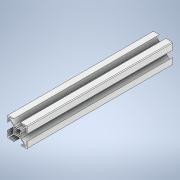
# Autodesk Inventor part: PerfilBaseJohan
Saved by Autodesk Inventor 2022.6 (Build 266554000, 554)
## iProperties
Created: 2025-01-14
Part Number: PerfilBaseJohan
Material: Genérico
Document SubType Name: Modeling
Designer: johan
Density: 1 g/cm^3
Appearance: Valor por defecto
Author: johan
Autodesk Inventor part; units mm, degrees
ref_plane "YZ Plane" through (0, 0, 0) normal (1, 0, 0) x (0, 1, 0)
ref_plane "XZ Plane" through (0, 0, 0) normal (0, 1, 0) x (-1, 0, 0)
ref_plane "XY Plane" through (0, 0, 0) normal (0, 0, 1) x (1, 0, 0)
sketch "Boceto1" plane through (0, 0, 0) normal (0, 0, 1) x (1, 0, 0)
  line L0 (0, 20) -> (7, 20)
  line L1 (7, 20) -> (7, 21)
  line L2 (0, 20) -> (1, 20)
  line L3 (1, 17.6407) -> (1, 15)
  line L4 (-1, 13) -> (0, 13)
  line L5 (5, 19) -> (2.3598, 19)
  arc A0 (5, 19) -> (6.7321, 20) centre (5, 21) ccw
  arc A1 (0, 13.2679) -> (1, 15) centre (-1, 15) ccw
  line L6 (20, 20) -> (13, 20)
  line L7 (19.3, 20) -> (19, 20)
  line L8 (19, 17.6402) -> (19, 15)
  line L9 (21, 13) -> (20, 13)
  line L10 (13, 20) -> (13, 21)
  line L11 (15, 19) -> (18.365, 19)
  arc A2 (13.2679, 20) -> (15, 19) centre (15, 21) ccw
  arc A3 (19, 15) -> (20, 13.2679) centre (21, 15) ccw
  line L12 (0.7, 0) -> (7, 0)
  line L13 (-1, 8.6378) -> (0, 8.6378)
  line L14 (7, 0) -> (7, -1)
  line L15 (5, 1) -> (2.3593, 1)
  line L16 (19.3, 0) -> (13, 0)
  line L17 (13, 0) -> (13, -1)
  line L18 (15, 1) -> (17.6402, 1)
  line L19 (19, 5) -> (19, 2.3593)
  arc A4 (20, 6.7321) -> (19, 5) centre (21, 5) ccw
  arc A5 (15, 1) -> (13.2679, 0) centre (15, -1) ccw
  arc A6 (6.7321, 0) -> (5, 1) centre (5, -1) ccw
  line L20 (20, 20) -> (13, 20)
  line L21 (7, 20) -> (0.7, 20)
  line L22 (0, 19.3) -> (0, 13)
  line L23 (0, 6.4641) -> (0, 0.7)
  line L24 (20, 0.7) -> (20, 6.7321)
  line L25 (20, 13) -> (20, 19.3)
  line L26 (0, 0) -> (7, 0)
  line L27 (13, 0) -> (20, 0)
  line L28 (17.6407, 19) -> (17.365, 19)
  line L29 (17.8529, 18.4879) -> (13.565, 14.2)
  line L30 (18.4883, 17.8528) -> (14.2, 13.5832)
  line L31 (1.5121, 17.8529) -> (5.8, 13.565)
  line L32 (2.1472, 18.4883) -> (6.4168, 14.2)
  line L33 (2.1471, 1.5121) -> (6.435, 5.8)
  line L34 (1.5117, 2.1472) -> (5.8, 6.4168)
  line L35 (18.4879, 2.1471) -> (14.2, 6.435)
  line L36 (17.8528, 1.5117) -> (13.5832, 5.8)
  line L37 (13, 13) -> (11.6766, 13.2679)
  line L38 (11.6766, 13.2679) -> (10.9786, 12.57)
  line L39 (13, 13) -> (13.2679, 11.6766)
  line L40 (13.2679, 11.6766) -> (12.57, 10.9786)
  line L41 (6.7321, 11.6766) -> (7.43, 10.9786)
  line L42 (7, 13) -> (6.7321, 11.6766)
  line L43 (7, 13) -> (8.3234, 13.2679)
  line L44 (8.3234, 13.2679) -> (9.0214, 12.57)
  line L45 (8.3234, 6.7321) -> (9.0214, 7.43)
  line L46 (7, 7) -> (8.3234, 6.7321)
  line L47 (7, 7) -> (6.7321, 8.3234)
  line L48 (6.7321, 8.3234) -> (7.43, 9.0214)
  line L49 (13.2679, 8.3234) -> (12.57, 9.0214)
  line L50 (13, 7) -> (13.2679, 8.3234)
  line L51 (13, 7) -> (11.6766, 6.7321)
  line L52 (11.6766, 6.7321) -> (10.9786, 7.43)
  line L53 (7, 13) -> (5.8, 14.2) construction
  line L54 (5.8, 5.8) -> (7, 7) construction
  line L55 (14.2, 5.8) -> (13, 7) construction
  line L56 (11.9445, 8.0555) -> (8.0555, 11.9445) construction
  line L57 (8.0555, 8.0555) -> (11.9445, 11.9445) construction
  line L58 (13, 13) -> (14.2, 14.2) construction
  arc A7 (10.9786, 12.57) -> (9.0214, 12.57) centre (10, 10) ccw
  arc A8 (12.57, 9.0214) -> (12.57, 10.9786) centre (10, 10) ccw
  arc A9 (7.43, 10.9786) -> (7.43, 9.0214) centre (10, 10) ccw
  arc A10 (9.0214, 7.43) -> (10.9786, 7.43) centre (10, 10) ccw
  line L59 (13.94, 10) -> (14.2, 10.9786)
  line L60 (13.94, 10) -> (14.2, 9.0214)
  line L61 (14.2, 6.435) -> (14.2, 9.0214)
  line L62 (14.2, 10.9786) -> (14.2, 13.5832)
  line L63 (10, 13.94) -> (10.9786, 14.2)
  line L64 (10.9786, 14.2) -> (10, 13.94)
  line L65 (10, 13.94) -> (9.0214, 14.2)
  line L66 (6.06, 10) -> (5.8, 10.9786)
  line L67 (6.06, 10) -> (5.8, 9.0214)
  line L68 (10, 6.06) -> (10.9786, 5.8)
  line L69 (10, 6.06) -> (9.0214, 5.8)
  line L70 (6.435, 5.8) -> (9.0214, 5.8)
  line L71 (10.9786, 5.8) -> (13.5832, 5.8)
  line L72 (5.8, 13.565) -> (5.8, 10.9786)
  line L73 (5.8, 9.0214) -> (5.8, 6.4168)
  line L74 (13.565, 14.2) -> (10.9786, 14.2)
  line L75 (9.0214, 14.2) -> (6.4168, 14.2)
  line L76 (1, 2.3598) -> (1, 4.7321)
  arc A11 (1, 4.7321) -> (0, 6.4641) centre (-1, 4.7321) ccw
  arc A12 (0.7, 20) -> (0, 19.3) centre (0.7, 19.3) ccw
  arc A13 (20, 19.3) -> (19.3, 20) centre (19.3, 19.3) ccw
  arc A14 (19.3, 0) -> (20, 0.7) centre (19.3, 0.7) ccw
  arc A15 (0, 0.7) -> (0.7, 0) centre (0.7, 0.7) ccw
  arc A16 (2.3598, 19) -> (2.1472, 18.4883) centre (2.3598, 18.7) ccw
  arc A17 (1.5121, 17.8529) -> (1, 17.6407) centre (1.3, 17.6407) ccw
  arc A18 (17.8529, 18.4879) -> (17.6407, 19) centre (17.6407, 18.7) ccw
  arc A19 (19, 17.6402) -> (18.4883, 17.8528) centre (18.7, 17.6402) ccw
  arc A20 (18.4879, 2.1471) -> (19, 2.3593) centre (18.7, 2.3593) ccw
  arc A21 (17.6402, 1) -> (17.8528, 1.5117) centre (17.6402, 1.3) ccw
  arc A22 (2.1471, 1.5121) -> (2.3593, 1) centre (2.3593, 1.3) ccw
  arc A23 (1, 2.3598) -> (1.5117, 2.1472) centre (1.3, 2.3598) ccw
  point P0 (7, 19)
  point P1 (1, 13)
  point P2 (19, 13)
  point P3 (1, 1.6378)
  point P4 (1, 8.6378)
  point P5 (7, 1)
  point P6 (13, 1)
  point P7 (19, 1.635)
  point P8 (1, 18.365)
  point P9 (19, 18.3622)
  point P10 (19.6406, 19)
  point P11 (1, 19.6406)
  point P12 (0.3594, 1)
  point P13 (19, 0.3594)
  point P14 (1.6378, 19)
  point P15 (1.635, 1)
  point P16 (18.3622, 1)
  dimension "d1" = 20
  dimension "d2" = 20
  dimension "d5" = 7
  dimension "d6" = 1
  dimension "d7" = 1
  dimension "d8" = 7
  dimension "d9" = 2
  dimension "d10" = 2
  dimension "d11" = 7
  dimension "d12" = 1
  dimension "d13" = 7
  dimension "d14" = 2
  dimension "d15" = 7
  dimension "d16" = 1
  dimension "d17" = 7
  dimension "d20" = 8.4
  dimension "d21" = 8.4
  dimension "d23" = 0.9
  dimension "d26" = 360
  dimension "d30" = 360
  dimension "d38" = 2
  dimension "d41" = 0.7
  dimension "d42" = 0.3
  constraints: 154 end point, 49 point on line, 48 point on circle, 38 tangent, 24 centre point, 23 perpendicular, 16 parallel, 12 equal radius, 5 horizontal, 2 midpoint, 1 collinear, 1 vertical, 66 other
  measures "d1" distance of L0.start L6.start
  measures "d2" distance of L6.start L27.end
  measures "d5" distance of L0.start L0.end
  measures "d6" distance of L0.end point (7, 19)
  measures "d7" distance of L0.start L2.end
  measures "d8" distance of L2.end point (1, 13)
  measures "d9" radius of A0
  measures "d10" radius of A1
  measures "d11" distance of L6.start L6.end
  measures "d12" distance of L6.start L7.end
  measures "d13" distance of L7.end point (19, 13)
  measures "d14" radius of A2
  measures "d15" distance of point (1, 1.638) point (1, 8.638)
  measures "d16" distance of L12.end point (7, 1)
  measures "d17" distance of L27.end L16.end
  measures "d20" distance of L53.end L58.end
  measures "d21" distance of L58.end L55.start
  measures "d23" distance of point (19, 18.362) L11.end
  measures "d38" radius of A11
  measures "d41" radius of A12
  measures "d42" radius of A16
extrude "Extrusión3" add sketch "Boceto1" against normal blind 146
